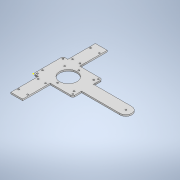
# Autodesk Inventor part: bottom_plate_impeller
Saved by Autodesk Inventor 2020 (Build 240168000, 168)
## iProperties
Created: 2023-05-22
Part Number: bottom_plate_impeller
Material: Типовые
Document SubType Name: Modeling
Designer: Администратор
Density: 1 g/cm^3
Appearance: По умолчанию
Author: Администратор
Autodesk Inventor part; units mm, degrees
ref_plane "YZ Plane" through (0, 0, 0) normal (1, 0, 0) x (0, 1, 0)
ref_plane "XZ Plane" through (0, 0, 0) normal (0, 1, 0) x (-1, 0, 0)
ref_plane "XY Plane" through (0, 0, 0) normal (0, 0, 1) x (1, 0, 0)
sketch "Эскиз1" plane through (0, 0, 0) normal (0, 1, 0) x (-1, 0, 0)
  line L0 (0, 0) -> (-80, 0) construction
  line L1 (-80, 0) -> (-80, -60) construction
  line L2 (-80, -60) -> (0, -60) construction
  line L3 (0, -60) -> (0, 0) construction
  line L4 (-4, -4) -> (-76, -4) construction
  line L5 (-76, -4) -> (-76, -56) construction
  line L6 (-76, -56) -> (-4, -56) construction
  line L7 (-4, -56) -> (-4, -4) construction
  circle A0 centre (-4, -4) radius 4 construction
  circle A1 centre (-4, -56) radius 4 construction
  circle A2 centre (-76, -56) radius 4 construction
  circle A3 centre (-76, -4) radius 4 construction
  line L8 (-76, -4) -> (-4, -56) construction
  line L9 (-4, -4) -> (-76, -56) construction
  line L10 (-40, -30) -> (-76, -30) construction
  line L11 (-76, -30) -> (-80, -30) construction
  line L12 (-80, -30) -> (-80, -42) construction
  line L13 (-80, -30) -> (-80, -18) construction
  line L14 (-80, -18) -> (-170, -18) construction
  line L15 (-170, -18) -> (-170, -42) construction
  line L16 (-170, -42) -> (-80, -42) construction
  line L17 (-80, -42) -> (-80, -18) construction
  line L18 (-80, -30) -> (-170, -30) construction
  line L19 (-170, -30) -> (-158, -30) construction
  circle A4 centre (-158, -30) radius 12 construction
  line L20 (0, 0) -> (-10, 0) construction
  line L21 (0, -60) -> (-10, -60) construction
  line L22 (0, 0) -> (-24, 0) construction
  line L23 (-10, 0) -> (-34, 0) construction
  line L24 (-34, 0) -> (-34, 56) construction
  line L25 (-34, 56) -> (-10, 56) construction
  line L26 (-10, 56) -> (-10, 0) construction
  line L27 (0, -60) -> (-10, -60) construction
  line L28 (-10, -60) -> (-34, -60) construction
  line L29 (-34, -60) -> (-34, -116) construction
  line L30 (-34, -116) -> (-10, -116) construction
  line L31 (-10, -116) -> (-10, -60) construction
  line L32 (0, -4) -> (0, -56)
  arc A5 (-4, -60) -> (0, -56) centre (-4, -56) ccw
  line L33 (-4, -60) -> (-10, -60)
  line L34 (-34, -116) -> (-10, -116)
  line L35 (-34, -60) -> (-76, -60)
  line L36 (-80, -56) -> (-80, -42)
  line L37 (-158, -42) -> (-80, -42)
  line L38 (-80, -18) -> (-158, -18)
  line L39 (-80, -18) -> (-80, -4)
  line L40 (-76, 0) -> (-34, 0)
  line L41 (-34, 0) -> (-34, 56)
  line L42 (-34, 56) -> (-10, 56)
  line L43 (-10, 56) -> (-10, 0)
  line L44 (-4, 0) -> (-10, 0)
  line L45 (-34, -60) -> (-34, -116)
  line L46 (-10, -60) -> (-10, -116)
  arc A6 (0, -4) -> (-4, 0) centre (-4, -4) ccw
  arc A7 (-76, 0) -> (-80, -4) centre (-76, -4) ccw
  arc A8 (-80, -56) -> (-76, -60) centre (-76, -56) ccw
  arc A9 (-158, -18) -> (-158, -42) centre (-158, -30) ccw
  circle A10 centre (-76, -56) radius 1.5
  circle A11 centre (-76, -4) radius 1.5
  circle A12 centre (-4, -4) radius 1.5
  circle A13 centre (-4, -56) radius 1.5
  circle A14 centre (-31, -103) radius 1.5
  circle A15 centre (-13, -103) radius 1.5
  line L47 (-31, -103) -> (-13, -103) construction
  circle A16 centre (-31, 43) radius 1.5
  circle A17 centre (-13, 43) radius 1.5
  line L48 (-31, 43) -> (-13, 43) construction
  line L49 (-22, -116) -> (-22, 56) construction
  circle A18 centre (-29.5, -65) radius 1.5
  circle A19 centre (-14.5, -65) radius 1.5
  line L50 (-29.5, -65) -> (-14.5, -65) construction
  circle A20 centre (-29.5, 5) radius 1.5
  circle A21 centre (-14.5, 5) radius 1.5
  line L51 (-29.5, 5) -> (-14.5, 5) construction
  circle A22 centre (-18.5, -45) radius 1.5
  circle A23 centre (-3.5, -15) radius 1.5
  circle A24 centre (-158, -30) radius 1.5
  circle A25 centre (-40.75, -30) radius 17.75
  circle A26 centre (-40.75, -51.75) radius 1.6
  circle A27 centre (-40.75, -8.25) radius 1.6
  line L52 (-80, -30) -> (-60, -30) construction
  line L53 (-18.5, -45) -> (-3.5, -15) construction
  line L54 (-1, -8.5) -> (-21, -8.5) construction
  line L55 (-21, -8.5) -> (-21, -51.5) construction
  line L56 (-21, -51.5) -> (-1, -51.5) construction
  line L57 (-1, -51.5) -> (-1, -8.5) construction
  line L58 (-1, -8.5) -> (-21, -51.5) construction
  line L59 (-21, -8.5) -> (-1, -51.5) construction
  line L60 (-65, -7) -> (-80, -7) construction
  line L61 (-80, -7) -> (-80, -53) construction
  line L62 (-80, -53) -> (-65, -53) construction
  line L63 (-65, -53) -> (-65, -7) construction
  line L64 (-72.5, -53) -> (-72.5, -7) construction
  circle A28 centre (-72.5, -50) radius 1.6
  line L65 (-72.5, -7) -> (-72.5, -53) construction
  circle A29 centre (-72.5, -10) radius 1.6
  line L66 (-59.9688, -15.5) -> (-112.9688, -15.5) construction
  line L67 (-112.9688, -15.5) -> (-112.9688, -44.5) construction
  line L68 (-112.9688, -44.5) -> (-59.9688, -44.5) construction
  line L69 (-59.9688, -44.5) -> (-59.9688, -15.5) construction
  point P0 (-11, -30)
  point P1 (-67.5382, -30)
  point P2 (-67.5382, -30)
  point P3 (-67.5382, -10)
  point P4 (-86.4688, -30)
  dimension "d3" = 80
  dimension "d4" = 60
  dimension "d5" = 72
  dimension "d6" = 52
  dimension "d7" = 4
  dimension "d8" = 4
  dimension "d9" = 8
  dimension "d10" = 8
  dimension "d11" = 8
  dimension "d12" = 8
  dimension "d13" = 12
  dimension "d14" = 12
  dimension "d15" = 90
  dimension "d16" = 24
  dimension "d17" = 12
  dimension "d18" = 10
  dimension "d21" = 24
  dimension "d22" = 56
  dimension "d23" = 24
  dimension "d24" = 56
  dimension "d27" = 3
  dimension "d28" = 3
  dimension "d29" = 3
  dimension "d30" = 3
  dimension "d31" = 3
  dimension "d32" = 3
  dimension "d33" = 18
  dimension "d34" = 13
  dimension "d35" = 3
  dimension "d36" = 3
  dimension "d37" = 3
  dimension "d38" = 15
  dimension "d39" = 5
  dimension "d44" = 3
  dimension "d45" = 3
  dimension "d46" = 30
  dimension "d47" = 15
  dimension "d48" = 15
  dimension "d52" = 3
  dimension "d55" = 35.5
  dimension "d56" = 40.75
  dimension "d57" = 3.2
  dimension "d58" = 21.75
  dimension "d59" = 20
  dimension "d60" = 20
  dimension "d61" = 43
  dimension "d62" = 15
  dimension "d63" = 46
  dimension "d65" = 3.5
  dimension "d68" = 3.2
  dimension "d69" = 3
  dimension "d70" = 0
  dimension "d71" = 53
  dimension "d72" = 29
  constraints: 140 end point, 30 centre point, 21 point on circle, 20 point on line, 16 parallel, 12 perpendicular, 11 midpoint, 10 coincident, 10 horizontal, 9 symmetric about line, 8 collinear, 5 tangent, 1 vertical, 6 other
  measures "d3" distance of L2.end L1.end
  measures "d4" distance of L1.end L0.end
  measures "d5" distance of L6.end L5.end
  measures "d6" distance of L5.end L4.end
  measures "d7" distance between parallel lines of L3 L7
  measures "d8" distance between parallel lines of L0 L4
  measures "d9" diameter of A0
  measures "d10" diameter of A1
  measures "d11" diameter of A2
  measures "d12" diameter of A3
  measures "d13" distance of L11.end L12.end
  measures "d14" distance of L11.end L13.end
  measures "d15" distance of L16.end L15.end
  measures "d16" distance of L15.end L14.end
  measures "d17" distance of L18.end L19.end
  measures "d18" distance of L0.start L20.end
  measures "d21" distance of L24.end L25.end
  measures "d22" distance of L23.end L24.end
  measures "d23" distance of L30.end L29.end
  measures "d24" distance of L29.end L28.end
  measures "d27" diameter of A10
  measures "d28" diameter of A11
  measures "d29" diameter of A12
  measures "d30" diameter of A13
  measures "d31" diameter of A14
  measures "d32" diameter of A15
  measures "d33" distance of L47.end L47.start
  measures "d34" distance from line of L30 L47.start
  measures "d35" distance from line of L47.start L29
  measures "d36" diameter of A18
  measures "d37" diameter of A19
  measures "d38" distance of L50.end L50.start
  measures "d39" distance from line of L50.start L2
  measures "d44" diameter of A22
  measures "d45" diameter of A23
  measures "d46" vertical distance of L53.end L53.start
  measures "d47" horizontal distance of L53.end L53.start
  measures "d48" distance from line of L0 L53.end
  measures "d52" diameter of A24
  measures "d55" diameter of A25
  measures "d56" distance from line of L32 A25.centre
  measures "d57" diameter of A26
  measures "d58" distance of A25.centre A26.centre
  measures "d59" distance of L11.end L52.end
  measures "d60" distance of L56.end L55.end
  measures "d61" distance of L55.end L54.end
  measures "d62" distance of L62.end L61.end
  measures "d63" distance of L61.end L60.end
  measures "d65" distance from line of L32 L53.end
  measures "d68" diameter of A28
  measures "d69" distance from line of L62 A28.centre
  measures "d70" distance between parallel lines of L1 L61
  measures "d71" distance of L68.end L67.end
  measures "d72" distance of L67.end L66.end
extrude "Выдавливание2" add sketch "Эскиз1" along normal blind 3
sketch "Эскиз2" plane through (0, 3, 0) normal (0, 1, 0) x (1, 0, 0)
  point P0 (0, 0)
